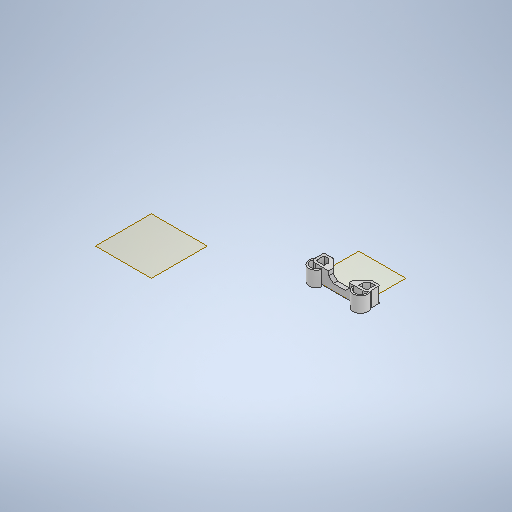
# Autodesk Inventor part: 20_Cube_4_insert_slideholder
Saved by Autodesk Inventor 2025.1 (Build 291241000, 241)
## iProperties
Created: 2024-10-07
Part Number: 20_Cube_4_insert_slideholder
Material: Generic
Document SubType Name: Modeling
Designer: diederichbenedict
Density: 1 g/cm^3
Appearance: Default
Author: diederichbenedict
Autodesk Inventor part; units mm, degrees
ref_plane "YZ Plane" through (0, 0, 0) normal (1, 0, 0) x (0, 1, 0)
ref_plane "XZ Plane" through (0, 0, 0) normal (0, 1, 0) x (-1, 0, 0)
ref_plane "XY Plane" through (0, 0, 0) normal (0, 0, 1) x (1, 0, 0)
ref_plane "Work Plane1" through (-277.443136, 66.349616, -144.544934) normal (0, 0, 1) x (-1, 0, 0)
ref_plane "Work Plane2" through (0, 0, 0) normal (0, 0, 1) x (1, 0, 0)
sketch "Sketch2" plane through (0, 0, 0) normal (0, 0, 1) x (1, 0, 0)
  line L0 (-14.02556, -18.096376) -> (14.02556, -18.096376)
  line L1 (-17, -21) -> (17, -21)
  line L2 (-17, -23.068589) -> (17, -23.068589)
  line L3 (17, -23.068589) -> (17, -21)
  line L4 (-17, -21) -> (17, -21)
  line L5 (-17, -21) -> (-17, -17)
  line L6 (-17, -17) -> (-21, -17)
  line L7 (-21, 17) -> (-21, -17)
  line L8 (-21, 17) -> (-23.485786, 17)
  line L9 (-23.485786, 17) -> (-23.485786, -17)
  line L10 (-23.485786, -17) -> (-24.9, -17)
  line L11 (-24.9, -17) -> (-24.9, -23.4)
  arc A0 (-24.9, -23.4) -> (-23.4, -24.9) centre (-23.4, -23.4) ccw
  line L12 (-23.4, -24.9) -> (-17, -24.9)
  line L13 (-17, -24.9) -> (-17, -23.068589)
  line L14 (-19.002607, -20.411607) -> (-18, -21.414214)
  line L15 (-18, -21.414214) -> (-18, -23.9)
  line L16 (-18, -23.9) -> (-23.4, -23.9)
  arc A1 (-23.9, -23.4) -> (-23.4, -23.9) centre (-23.4, -23.4) ccw
  line L17 (-23.9, -23.4) -> (-23.9, -18)
  line L18 (-23.9, -18) -> (-21.414214, -18)
  line L19 (-21.414214, -18) -> (-20.411607, -19.002607)
  arc A2 (-19.002607, -20.411607) -> (-20.411607, -19.002607) centre (-20.5, -20.5) ccw
  line L20 (-17, -21) -> (-21, -17)
  line L21 (17.1, -21) -> (17.1, -23.168589)
  line L22 (17.1, -23.168589) -> (-16.9, -23.168589)
  line L23 (-16.9, -23.168589) -> (-16.9, -25)
  line L24 (-16.9, -25) -> (-23.4, -25)
  arc A3 (-25, -23.4) -> (-23.4, -25) centre (-23.4, -23.4) ccw
  line L25 (-25, -23.4) -> (-25, -16.9)
  line L26 (-25, -16.9) -> (-23.585786, -16.9)
  line L27 (-23.585786, -16.9) -> (-23.585786, 17.1)
  line L28 (-23.585786, 17.1) -> (-20.9, 17.1)
  line L29 (-20.9, 17.1) -> (-20.9, -16.9)
  line L30 (-18.518494, -17) -> (-18.518494, 19.481506)
  line L31 (-18.518494, 19.481506) -> (-25.967293, 19.481506)
  line L32 (-25.967293, 19.481506) -> (-25.967293, -14.518494)
  line L33 (-25.967293, -14.518494) -> (-27.381506, -14.518494)
  line L34 (-27.381506, -14.518494) -> (-27.381506, -23.4)
  arc A4 (-27.381506, -23.4) -> (-23.4, -27.381506) centre (-23.4, -23.4) ccw
  line L35 (-23.4, -27.381506) -> (-14.518494, -27.381506)
  line L36 (-14.518494, -27.381506) -> (-14.518494, -25.550095)
  line L37 (-14.518494, -25.550095) -> (19.481506, -25.550095)
  line L38 (19.481506, -25.550095) -> (19.481506, -21)
  line L39 (-25.967293, -14.518494) -> (-18.518494, -14.518494)
  line L40 (-18.518494, -14.518494) -> (-9.968398, -23.068589)
  line L41 (-9.968398, -23.068589) -> (-9.968398, -27.381506)
  line L42 (-9.968398, -27.381506) -> (-14.518494, -27.381506)
  line L43 (-25, -14.518494) -> (-25, -16.9)
  line L44 (-23.585786, -16.9) -> (-20.9, -16.9)
  line L45 (-16.9, -23.168589) -> (-16.9, -21.1)
  line L46 (-16.9, -21.1) -> (-20.9, -16.9)
  line L47 (0, -22.303314) -> (0, -14.676159)
  line L48 (-16.9, -25) -> (0, -25)
  line L49 (0, -25) -> (0, -17)
  line L50 (0, -17) -> (-16.9, -17)
  line L51 (-16.9, -17) -> (-16.9, -25)
  line L52 (-14.808037, -27.381506) -> (0, -27.381506)
  line L53 (0, -27.381506) -> (0, -23.168589)
  line L54 (0, -23.168589) -> (-14.808037, -23.168589)
  line L55 (-14.808037, -23.168589) -> (-14.808037, -27.381506)
  arc A5 (-26.848471, -25.390085) -> (-16.085212, -28.681506) centre (-21.698424, -27.793091) ccw
  arc A6 (-27.381506, -23.4) -> (-14.570493, -28.681506) centre (-21.698424, -27.793091) ccw
  line L56 (-16.085212, -28.681506) -> (-14.570493, -28.681506)
  point P0 (0, 0)
  point P1 (-20.15, -25)
  point P2 (-25.365623, -26.862473)
  point P3 (-23.656712, -24.979272)
  point P4 (-23.585786, -14.518494)
  point P5 (-23.485786, -16.9)
  point P6 (-21, -16.9)
  point P7 (-21, -14.518494)
  point P8 (-23.485786, -14.518494)
  point P9 (-9.968398, -25.550095)
  point P10 (-9.968398, -25)
  point P11 (-16.9, -21)
  point P12 (-16.9, -23.068589)
  point P13 (0, -23.068589)
  point P14 (-16.036987, -17)
  point P15 (-20.9, -14.518494)
  point P16 (-16.995238, -21)
  point P17 (0, -25)
  point P18 (-9.968398, -23.168589)
  dimension "d0" = 0.1
  dimension "d1" = 2.38151
  dimension "d11" = 1.5
  dimension "d12" = 1.3
  constraints: 72 end point, 12 point on circle, 8 point on line, 6 perpendicular, 5 parallel, 4 centre point, 3 vertical, 2 horizontal, 1 coincident, 1 midpoint, 1 tangent, 18 other
  measures "d0" distance from line of point (-20.15, -25) L12
  measures "d1" distance between parallel lines of L26 L33
  measures "d11" radial gap between concentric circles of A6 A5
  measures "d12" distance between parallel lines of L56 L35
extrude "Extrusion1" add sketch "Sketch2" along normal blind 15 contours L46 L5 L6 L30 L40 L50 L51 L1 | L46 L6 L5 | L51 L50 L40 L1 | L1 L40 L2 L45 L51 | L46 L29 L39 L30 L6 | L44 L9 L39 L7 | L7 L39 L29 L44 | L2 L41 L22 L45 | L44 L27 L39 L9 | L22 L55 L48 L23 | L26 L43 L39 L27 | L41 L48 L55 L22 | L22 L49 L48 L41 | L48 L55 L35 A4 L34 L33 L39 L43 L25 A3 L24 | L48 L53 L37 L41 | L41 L37 L36 L35 L55 L48 | L41 L42 L36 L37 | L37 L53 L52 L41 | A5 L56 A6 A4
mirror "Mirror1" about plane through (0, -27.381506, 0) normal (1, 0, 0) of "Extrusion1"
fillet "Fillet1" radius 1 12 edges at (-14.5705, -28.6815, 7.5) (-18.5185, -14.5185, 7.5) (-27.3815, -14.5185, 7.5) (-9.9684, -23.0686, 7.5) (9.9684, -23.0686, 7.5) (18.5185, -14.5185, 7.5) (27.3815, -14.5185, 7.5) (27.3815, -23.4, 7.5) (-27.3815, -23.4, 7.5) (14.5705, -28.6815, 7.5) (-16.0852, -28.6815, 7.5) (16.0852, -28.6815, 7.5)
sketch "Skizze3" plane through (-23.4, -27.381506, 0) normal (0, -1, 0) x (1, 0, 0)
  line L0 (0, 0) -> (46.8, 0)
  line L1 (46.8, 0) -> (46.8, 15)
  line L2 (0, 15) -> (46.8, 15)
  line L3 (0, 0) -> (0, 15)
  line L4 (13.431602, 0) -> (13.431602, 15)
  line L5 (0, 15) -> (46.8, 15)
  line L6 (33.368398, 0) -> (33.368398, 15)
  line L7 (9.370625, 15) -> (17.855906, 6.514719)
  line L8 (9.370625, 15) -> (21.370625, 15) construction
  line L9 (38.258557, 15) -> (52.281506, 15)
  line L10 (38.258557, 0) -> (38.258557, 15)
  line L11 (38.258557, 15) -> (29.773276, 6.514719)
  line L12 (38.258557, 15) -> (50.258557, 15) construction
  line L13 (29.773276, 6.514719) -> (17.855906, 6.514719)
  point P0 (23.4, 0)
  point P1 (50.964811, 15)
  point P2 (33.368398, 10.109841)
  point P3 (13.431602, 10.939023)
  dimension "d13" = 12
  dimension "d14" = 45
  dimension "d15" = 135
  constraints: 10 end point, 3 horizontal, 2 equal length, 1 point on line
  measures "d13" distance of L7.start L7.end
  measures "d14" angle of L7 L8
  measures "d15" angle of L11 L12
extrude "Extrusion2" cut sketch "Skizze3" against normal blind 15 contours L4 L2 L6 L11 L13 L7
body "Solid1"
